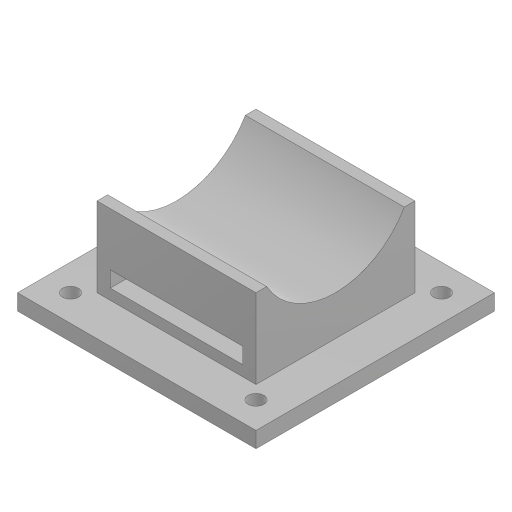
# Autodesk Inventor part: fastening-clip
Saved by Autodesk Inventor 2023.1 (Build 271208000, 208)
## iProperties
Created: 2022-08-30
Part Number: fastening-clip
Material: PC/ABS-Kunststoff
Document SubType Name: Modeling
Designer: tland
Density: 0.357273 g/cm^3
Appearance: Glatt - Mittelgrau
Author: tland
Autodesk Inventor part; units mm, degrees
ref_plane "YZ Plane" through (0, 0, 0) normal (1, 0, 0) x (0, 1, 0)
ref_plane "XZ Plane" through (0, 0, 0) normal (0, 1, 0) x (-1, 0, 0)
ref_plane "XY Plane" through (0, 0, 0) normal (0, 0, 1) x (1, 0, 0)
sketch "Skizze1" plane through (0, 0, 0) normal (0, 1, 0) x (-1, 0, 0)
  line L0 (22.5, 22.5) -> (-22.5, 22.5)
  line L1 (-22.5, 22.5) -> (-22.5, -22.5)
  line L2 (-22.5, -22.5) -> (22.5, -22.5)
  line L3 (22.5, -22.5) -> (22.5, 22.5)
  line L4 (17.5, 17.5) -> (-17.5, 17.5) construction
  line L5 (-17.5, 17.5) -> (-17.5, -17.5) construction
  line L6 (-17.5, -17.5) -> (17.5, -17.5) construction
  line L7 (17.5, -17.5) -> (17.5, 17.5) construction
  circle A0 centre (17.5, 17.5) radius 1.5
  circle A1 centre (17.5, -17.5) radius 1.5
  circle A2 centre (-17.5, 17.5) radius 1.5
  circle A3 centre (-17.5, -17.5) radius 1.5
  point P0 (0, 0)
  point P1 (0, 22.5)
  point P2 (22.5, 0)
  dimension "d0" = 45
  dimension "d1" = 5
  dimension "d2" = 35
  dimension "d3" = 3
  constraints: 16 end point, 4 centre point, 4 coincident, 4 parallel, 3 equal radius, 3 perpendicular, 2 midpoint, 1 horizontal, 1 horizontal alignment, 1 vertical alignment, 3 other
  measures "d0" distance of L2.end L0.start
  measures "d1" distance between parallel lines of L3 L7
  measures "d2" distance of L6.end L4.start
  measures "d3" diameter of A0
extrude "Extrusion1" add sketch "Skizze1" along normal blind 3
sketch "Skizze2" plane through (0, 3, 0) normal (0, 1, 0) x (1, 0, 0)
  line L0 (-15, -15) -> (15, -15)
  line L1 (15, -15) -> (15, 15)
  line L2 (15, 15) -> (-15, 15)
  line L3 (-15, 15) -> (-15, -15)
  point P0 (0, 0)
  point P1 (0, -15)
  point P2 (-15, 0)
  dimension "d7" = 30
  constraints: 8 end point, 2 midpoint, 2 parallel, 2 perpendicular, 1 horizontal, 1 horizontal alignment, 1 vertical alignment
  measures "d7" distance of L2.end L0.start
extrude "Extrusion2" add sketch "Skizze2" along normal blind 30
sketch "Skizze3" plane through (15, 3, 15) normal (1, 0, 0) x (0, 0, -1)
  circle A0 centre (15, 22.5) radius 15
  line L0 (-7.5, 0) -> (37.5, 0) construction
  line L1 (-7.5, -3) -> (37.5, -3) projected
  point P0 (15, -3)
  point P1 (15, -3)
  point P2 (15, 0)
  point P3 (15, 7.5)
  point P4 (15, 0)
  point P5 (15, -3)
  dimension "d10" = 30
  dimension "d18" = 7.5
  constraints: 4 midpoint, 3 vertical alignment, 2 other
  measures "d18" distance of point (15, 7.5) point (15, 0)
extrude "Extrusion3" cut sketch "Skizze3" against normal through all
sketch "Skizze4" plane through (15, 3, -15) normal (1, 0, 0) x (0, 0, -1)
  line L0 (0, 30) -> (-30, 30)
  line L1 (-30, 30) -> (-30, 15)
  line L2 (-30, 15) -> (0, 15)
  line L3 (0, 15) -> (0, 30)
  arc A0 (-27.9904, 30) -> (-2.0096, 30) centre (-15, 22.5) ccw construction
  point P0 (-15, -3)
  point P1 (-15, 0)
  dimension "d24" = 15
  constraints: 8 end point, 2 parallel, 1 coincident, 1 horizontal, 1 perpendicular, 1 other
  measures "d24" distance of L2.end L0.start
extrude "Extrusion4" cut sketch "Skizze4" against normal through all
sketch "Skizze5" plane through (15, 3, -15) normal (0, 0, -1) x (-1, 0, 0)
  line L0 (27.5, 5) -> (2.5, 5)
  line L1 (2.5, 5) -> (2.5, 2)
  line L2 (2.5, 2) -> (27.5, 2)
  line L3 (27.5, 2) -> (27.5, 5)
  line L4 (-7.5, 0) -> (37.5, 0) construction
  point P0 (15, -3)
  point P1 (15, 2)
  dimension "d19" = 25
  dimension "d20" = 3
  dimension "d21" = 2
  constraints: 8 end point, 2 parallel, 1 horizontal, 1 midpoint, 1 perpendicular, 1 vertical alignment
  measures "d19" distance of L0.start L0.end
  measures "d20" distance of L2.end L0.start
  measures "d21" distance between parallel lines of L4 L2
extrude "Extrusion5" cut sketch "Skizze5" against normal through all
